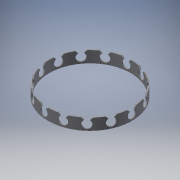
# Autodesk Inventor part: cage
Saved by Autodesk Inventor 2017 (Build 210142000, 142)
## iProperties
Created: 2017-12-10
Part Number: cage
Material: Generic
Document SubType Name: Modeling
Designer: prakhar
Density: 1 g/cm^3
Appearance: Default
Author: prakhar
Autodesk Inventor part; units mm, degrees
ref_plane "YZ Plane" through (0, 0, 0) normal (1, 0, 0) x (0, 1, 0)
ref_plane "XZ Plane" through (0, 0, 0) normal (0, 1, 0) x (-1, 0, 0)
ref_plane "XY Plane" through (0, 0, 0) normal (0, 0, 1) x (1, 0, 0)
sketch "Sketch1" plane through (0, 0, 0) normal (0, 1, 0) x (-1, 0, 0)
  circle A0 centre (0, 0) radius 46.736
  circle A1 centre (0, 0) radius 45.339
  dimension "d0" = 93.472
  dimension "d1" = 90.678
  constraints: 2 centre point, 2 coincident
  measures "d0" diameter of A0
  measures "d1" diameter of A1
extrude "Extrusion1" add sketch "Sketch1" along normal blind 12.7
sketch "Sketch2" plane through (0, 0, 0) normal (1, 0, 0) x (0, 1, 0)
  circle A0 centre (6.35, 0) radius 3.81
  point P0 (0, 0)
  dimension "d4" = 7.62
  dimension "d5" = 6.35
  constraints: 1 centre point
  measures "d4" diameter of A0
  measures "d5" distance of A0.centre point (0, 0)
extrude "Extrusion2" cut sketch "Sketch2" along normal blind 77.7875
sketch "Sketch3" plane through (0, 0, 0) normal (1, 0, 0) x (0, 1, 0)
  arc A0 (9.339, 3.29) -> (6.8803, 4.4133) centre (6.35, 0) ccw
  line L0 (12.7, 45.339) -> (12.7, -45.339) projected
  line L1 (12.7, 4.9779) -> (10.1034, 2.3813)
  line L2 (0, -45.339) -> (0, 45.339) projected
  line L3 (12.7, -46.736) -> (12.7, 46.736) projected
  line L4 (0, 0) -> (1.905, 0)
  line L5 (10.795, 0) -> (12.7, 0)
  line L6 (10.795, 0) -> (6.995, 0)
  line L7 (6.995, 0) -> (6.995, 2.3812)
  line L8 (6.995, 2.3812) -> (10.1034, 2.3813)
  line L9 (10.795, 2.3813) -> (10.795, 0)
  arc A1 (6.8803, 4.4133) -> (10.1034, 2.3813) centre (6.35, 0) ccw
  line L10 (12.7, 4.9779) -> (12.7, 0)
  arc A2 (10.1034, 2.3813) -> (9.339, 3.29) centre (6.35, 0) ccw
  line L11 (10.1034, 2.3813) -> (10.795, 2.3813)
  dimension "d8" = 8.89
  dimension "d9" = 6.35
  dimension "d11" = 45
  dimension "d14" = 2.3813
  dimension "d21" = 2.032
  constraints: 18 end point, 9 point on circle, 3 centre point, 3 horizontal, 3 horizontal alignment, 3 parallel, 2 midpoint, 2 perpendicular, 2 point on line
  measures "d8" diameter of A0
  measures "d9" distance of A0.centre point (0, 0)
  measures "d11" angle of L0 L1
  measures "d14" vertical distance of L1.end A0.centre
  measures "d21" vertical distance of L1.end A0.end
extrude "Extrusion5" cut sketch "Sketch3" along normal blind 77.7875
mirror "Mirror3" about plane through (0, 0, 0) normal (0, 0, 1) of "Extrusion5"
pattern_circular "Circular Pattern1" count 15 over 360 about axis through (0, -10, 0) along (0, 1, 0) of "Extrusion2", "Extrusion5", "Mirror3"
body "Solid1"
